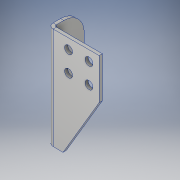
# Autodesk Inventor part: Roller bracket
Saved by Autodesk Inventor 2019 (Build 230136000, 136)
## iProperties
Created: 2018-11-09
Part Number: Roller bracket
Material: Aluminum 6061
Document SubType Name: Sheet Metal
Designer: woodk
Density: 2.7 g/cm^3
Sheet Metal Rule: Haakon
Appearance: Aluminum - Flat
Mass: 13.7005 g
Surface Area: 55.719 cm^2
Volume: 5.07426 cm^3
Author: woodk
Autodesk Inventor part; units mm, degrees
note: some values were not read from the file. Chosen so that the rebuilt part matches the saved one: flange form of "Plate2".
ref_plane "YZ Plane" through (0, 0, 0) normal (1, 0, 0) x (0, 1, 0)
ref_plane "XZ Plane" through (0, 0, 0) normal (0, 1, 0) x (-1, 0, 0)
ref_plane "XY Plane" through (0, 0, 0) normal (0, 0, 1) x (1, 0, 0)
sketch "Sketch1" plane through (0, 0, 0) normal (0, 0, 1) x (1, 0, 0)
  line L0 (0, 0) -> (32.0167, 0)
  line L1 (32.0167, 0) -> (32.0167, 63.5)
  line L2 (32.0167, 63.5) -> (0, 63.5)
  line L3 (0, 63.5) -> (0, 0)
  dimension "d0" = 63.5
  dimension "d1" = 32.0167
  measures "d0" distance of L2.end L0.start
  measures "d1" distance of L0.start L0.end
extrude "Plate1" add sketch "Sketch1" along normal blind 2.032
sketch "Sketch2" plane through (2.032, 63.5, 2.032) normal (-1, 0, 0) x (0, -1, 0)
  line L0 (63.5, 0) -> (0, 0)
  line L1 (0, 0) -> (0, -20.6375)
  line L2 (0, -20.6375) -> (63.5, -20.6375)
  line L3 (63.5, -20.6375) -> (63.5, 0)
  constraints: 6 end point, 1 horizontal, 1 perpendicular, 1 vertical
edge flange "Flange1" height 20.6375 angle 90 thickness 2.032 bend radius 1.27 thickness toward (-1, 0, 0) relief tear relief width 2.032 relief depth 1.016 edges at (0, 31.75, 0) wall of the first edge with corners at (2.032, 0, 2.032) (2.032, 63.5, 2.032) (2.032, 63.5, -18.6055) (2.032, 0, -18.6055)
bend "Bend1"
corner "Corner1"
sketch "Sketch3" plane through (0, 0, 0) normal (0, 0, -1) x (-1, 0, 0)
  line L0 (-32.0167, 0) -> (-32.0167, 63.5) projected
  line L1 (-32.0167, 63.5) -> (-3.302, 63.5) projected
  point P0 (0, 0)
  point P1 (-25.6667, 57.15)
  point P2 (-12.9667, 57.15)
  point P3 (-25.6667, 44.45)
  point P4 (-12.9667, 44.45)
  dimension "d13" = 6.35
  dimension "d14" = 6.35
  dimension "d15" = 12.7
  dimension "d16" = 12.7
  constraints: 2 horizontal alignment, 2 vertical alignment
  measures "d13" distance from line of L0 point (-25.667, 57.15)
  measures "d14" distance from line of L1 point (-25.667, 57.15)
  measures "d15" distance of point (-25.667, 57.15) point (-25.667, 44.45)
  measures "d16" distance of point (-25.667, 57.15) point (-12.967, 57.15)
hole "Hole1" at (25.6667, 57.15, 0) at (12.9667, 57.15, 0) at (25.6667, 44.45, 0) at (12.9667, 44.45, 0) direction (0, 0, 1) diameter 4.9784 end through all
sketch "Sketch4" plane through (2.032, 0, -18.6055) normal (1, 0, 0) x (0, 0, -1)
  line L0 (-20.6375, 63.5) -> (-20.6375, 0) projected
  line L1 (-17.3355, 0) -> (0, 0) projected
  point P0 (-18.6055, 0)
  point P1 (-7.9375, 7.62)
  dimension "d31" = 12.7
  dimension "d32" = 7.62
  measures "d31" distance from line of L0 point (-7.938, 7.62)
  measures "d32" distance from line of L1 point (-7.938, 7.62)
hole "Hole2" at (2.032, 7.62, -10.668) direction (-1, 0, 0) diameter 6.35 end through all clearance for "Flat Head Machine Screw (82)" size "1/4" standard "Ansi Unified Screw Threads"
fillet "Fillet1" radius 12.7 1 edges at (1.016, 63.5, -18.6055)
sketch "Sketch5" plane through (0, 0, 0) normal (0, 0, -1) x (-1, 0, 0)
  line L0 (-32.0167, 38.1) -> (-9.525, 0)
  line L1 (-32.0167, 0) -> (-3.302, 0) projected
  line L2 (0, 0) -> (0, 50.8) projected
  line L3 (-32.0167, 63.5) -> (-3.302, 63.5) projected
  line L4 (-32.0167, 0) -> (-32.0167, 63.5) projected
  line L5 (-32.0167, 38.1) -> (-32.0167, 0)
  line L6 (-32.0167, 0) -> (-9.525, 0)
  dimension "d34" = 9.525
  dimension "d35" = 25.4
  constraints: 6 end point, 2 point on line, 1 perpendicular, 1 vertical
  measures "d34" distance from line of L2 L0.end
  measures "d35" distance from line of L3 L0.start
extrude "Extrusion1" cut sketch "Sketch5" against normal through all
equation "\"d22\" = Thickness"
equation "\"d29\" = Thickness"
equation "\"d2\" = Thickness"
equation "\"d3\" = BendReliefWidth"
equation "\"d4\" = BendReliefDepth"
equation "\"d5\" = MinimumRemnant"
equation "\"d6\" = TransitionRadius"
equation "\"d9\" = BendRadius"
equation "\"d10\" = CornerReliefSize"
equation "\"d11\" = GapSize"
equation "\"d12\" = JacobiRadiusSize"
equation "\"BendReliefWidth\" = Thickness"
equation "\"BendReliefDepth\" = 0.5 * Thickness"
equation "\"CornerReliefSize\" = 4 * Thickness"
equation "\"MinimumRemnant\" = 2 * Thickness"
equation "\"TransitionRadius\" = BendRadius"
equation "\"JacobiRadiusSize\" = BendRadius"
equation "\"GapSize\" = Thickness"
equation "\"Thickness\" = 2.032"
equation "\"BendRadius\" = 1.27"
body "Solid1"
